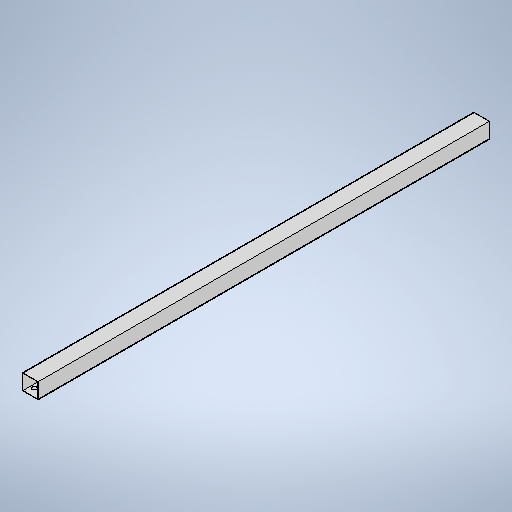
# Autodesk Inventor part: DMF 082 коллектор болванка
Saved by Autodesk Inventor 2026.2 (Build 302298010, 298A)
## iProperties
Created: 2024-06-28
Part Number: DMF 082 коллектор болванка
Material: Generic
Document SubType Name: Modeling
Designer: admin
Density: 1 g/cm^3
Appearance: Default
Author: admin
Autodesk Inventor part; units mm, degrees
ref_plane "YZ Plane" through (0, 0, 0) normal (1, 0, 0) x (0, 1, 0)
ref_plane "XZ Plane" through (0, 0, 0) normal (0, 1, 0) x (-1, 0, 0)
ref_plane "XY Plane" through (0, 0, 0) normal (0, 0, 1) x (1, 0, 0)
sketch "Sketch2" plane through (0, 0, 0) normal (0, 1, 0) x (-1, 0, 0)
  line L0 (40, 40) -> (-40, 40)
  line L1 (-40, 40) -> (-40, -40)
  line L2 (-40, -40) -> (40, -40)
  line L3 (40, -40) -> (40, 40)
  line L4 (40, 40) -> (-40, -40) construction
  line L5 (-40, 40) -> (40, -40) construction
  line L6 (-38, -38) -> (-38, 38)
  line L7 (-38, 38) -> (38, 38)
  line L8 (38, 38) -> (38, -38)
  line L9 (38, -38) -> (-38, -38)
  point P0 (0, 0)
  point P1 (0, -190)
  point P2 (0, 0)
  dimension "d6" = 80
  dimension "d49" = 2
  constraints: 20 end point, 4 parallel, 3 perpendicular, 2 midpoint, 1 coincident, 1 horizontal, 3 other
  measures "d6" distance of L2.end L0.start
  measures "d49" distance between parallel lines of L1 L6
extrude "Extrusion2" add sketch "Sketch2" along normal blind 2300
sketch "Sketch6" plane through (40, 0, -40) normal (0, 0, -1) x (-1, 0, 0)
  line L0 (0, 0) -> (80, 0) projected
  line L1 (80, 0) -> (80, 2300) construction
  line L2 (0, 2300) -> (80, 2300)
  line L3 (0, 0) -> (0, 2300) construction
  circle A0 centre (60, 40) radius 10.75
  circle A1 centre (20, 360) radius 10.75
  point P0 (40, 0)
  dimension "d44" = 21.5
  dimension "d45" = 20
  dimension "d46" = 20
  dimension "d47" = 320
  dimension "d48" = 40
  constraints: 2 centre point, 2 end point, 1 equal radius
  measures "d44" diameter of A0
  measures "d45" distance from line of L1 A0.centre
  measures "d46" distance from line of A1.centre L3
  measures "d47" vertical distance of A1.centre A0.centre
  measures "d48" distance from line of A0.centre L0
extrude "Extrusion6" cut sketch "Sketch6" against normal up to surface (2 mm away)
equation "\"d46\" = d45"
body "Solid2"
